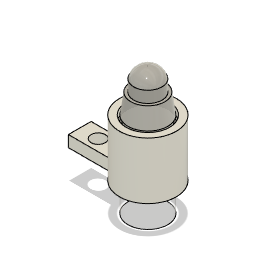
RGB General Illumination Light (Autodesk Fusion 360 design; units mm, degrees)
Autodesk Fusion 360 part; units mm, degrees
note: some values were not read from the file. Set by a fixed rule: which sketch regions a step uses.
sketch "Sketch1" plane through (0, 0, 0) normal (0, 1, 0) x (1, 0, 0) in component "GI Socket"
  circle A0 centre (0, 0) radius 7.9375
  circle A1 centre (0, 0) radius 6.5
  circle A2 centre (0, 0) radius 6.05
  line L0 (-19.05, 3.175) -> (-7.2748, 3.175)
  line L1 (-19.05, 3.175) -> (-19.05, -3.175)
  line L2 (-19.05, -3.175) -> (-7.2748, -3.175)
  circle A3 centre (-13.8906, 0) radius 1.9844
  dimension "d1" = 15.875
  dimension "d2" = 13
  dimension "d3" = 12.1
  dimension "d5" = 3.9688
  constraint coincident A0.centre A1.centre
  constraint concentric A0 A1
  constraint concentric A1 A2
  constraint coincident A0 L0.end
  constraint horizontal L0
  constraint perpendicular L0 L1
  constraint coincident A0 L2.end
  constraint perpendicular L1 L2
  measures "d1" diameter of A0
  measures "d2" diameter of A1
  measures "d3" diameter of A2
  measures "d5" diameter of A3
extrude "Extrude1" add sketch "Sketch1" along normal blind 3.175 contours A0 L0 L1 L2 makes body 1 in component "GI Socket"
extrude "Extrude2" add sketch "Sketch1" along normal blind 15.875 contours A0 | A1 bodies 1 in component "GI Socket"
extrude "Extrude3" cut sketch "Sketch1" along normal blind 13.97 contours A1 bodies 1 in component "GI Socket"
copy_body "CutPasteBodies1" bodies 1 removing the originals makes body 2 in component "GI Socket"
sketch "Sketch1 (2)" plane through (0, 0, 0) normal (0, 0, 1) x (1, 0, 0) in component "GI Bulb"
  line L0 (25.4, 0) -> (30.9562, 0)
  line L1 (30.9562, 0) -> (30.9562, 22.225)
  line L2 (30.9562, 22.225) -> (30.5594, 22.225)
  line L3 (30.5594, 22.225) -> (30.5594, 23.8125)
  line L4 (30.5594, 23.8125) -> (30.9562, 23.8125)
  line L5 (29.3687, 29.3688) -> (29.3687, 32.5438)
  line L6 (25.4, 35.7188) -> (25.4254, 35.7188)
  line L7 (29.3687, 32.5438) -> (29.3687, 32.5701)
  line L8 (25.4, 35.7188) -> (25.4, 0)
  arc A0 (29.3687, 32.5701) -> (25.4254, 35.7188) centre (25.4254, 31.6751) ccw
  line L9 (29.3687, 29.3688) -> (30.1625, 29.3688)
  line L10 (30.9562, 23.8125) -> (30.1625, 29.3688)
  point P0 (25.4, 0.7937)
  dimension "d12" = 5.5563
  dimension "d13" = 22.225
  dimension "d14" = 0.3969
  dimension "d15" = 1.5875
  dimension "d16" = 0.3969
  dimension "d20" = 3.175
  dimension "d23" = 0.0254
  dimension "d24" = 0.0264
  dimension "d34" = 0.7937
  constraint horizontal L0
  constraint perpendicular L0 L1
  constraint horizontal L2
  constraint perpendicular L2 L3
  constraint perpendicular L3 L4
  constraint horizontal L6
  constraint perpendicular L0 L8
  constraint coincident L8 P0
  constraint tangent L6 A0
  constraint horizontal L9
  measures "d12" distance of L0.start L0.end
  measures "d13" distance of L0.end L1.end
  measures "d14" distance of L1.end L2.end
  measures "d15" distance of L2.end L3.end
  measures "d16" distance of L3.end L4.end
  measures "d20" distance of L5.start L5.end
  measures "d23" distance of L6.start L6.end
  measures "d34" distance of L5.start L9.end
sketch "Sketch2" plane through (0, 0, 0) normal (0, 1, 0) x (1, 0, 0) in component "GI Bulb"
  circle A0 centre (25.4, 0) radius 5.5563
  point P0 (25.4, 0)
  dimension "d25" = 11.1125
  constraint coincident P0 A0.centre
  measures "d25" diameter of A0
sweep "Sweep1" add profiles "Sketch1 (2)" path "Sketch2" along A0 section 1 separate body makes body 3 in component "GI Bulb"
component "GI Socket" placed x (1, 0, 0) y (0, 1, 0) z (0, 0, 1) at (0, 0, 0)
component "GI Bulb" placed x (1, 0, 0) y (0, 1, 0) z (0, 0, 1) at (-25.4, -7.9375, 0)
equation "d5 = ( 5 / 32 ) * 1 in"
equation "d6 = ( 1 / 8 ) * 1 in"
equation "d8 = ( 5 / 8 ) * 1 in"
equation "d12 = ( 7 / 32 ) * 1 in"
equation "d13 = ( 7 / 8 ) * 1 in"
equation "d14 = ( 1 / 64 ) * 1 in"
equation "d15 = ( 1 / 16 ) * 1 in"
equation "d16 = ( 1 / 64 ) * 1 in"
equation "d20 = ( 1 / 8 ) * 1 in"
equation "d25 = ( 7 / 16 ) * 1 in"
equation "d34 = ( 1 / 32 ) * 1 in"
